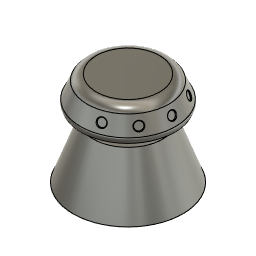
forme1 (Autodesk Fusion 360 design; units mm, degrees)
Autodesk Fusion 360 part; units mm, degrees
note: some values were not read from the file. Set by a fixed rule: which sketch regions a step uses.
sketch "Esquisse2" plane through (0, 0, 0) normal (0, 0, 1) x (1, 0, 0)
  line L0 (-70, 0) -> (-98.2998, 28.2688)
  line L1 (-98.2998, 28.2688) -> (-76.4677, 78.2688)
  line L2 (-76.4677, 78.2688) -> (0, 78.2688)
  line L3 (0, 78.2688) -> (0, 0)
  line L4 (-70, 0) -> (-110, -110)
  line L5 (-110, -110) -> (0, -110)
  line L6 (0, -110) -> (0, 0)
  dimension "d4" = 40
  dimension "d5" = 70
  dimension "d6" = 50
  dimension "d12" = 110
  constraint horizontal L2
  constraint coincident L3.end L6.end
  measures "d4" distance of L0.start L0.end
  measures "d5" distance of L3.end L0.start
  measures "d6" vertical distance of L0.end L1.end
  measures "d12" vertical distance of L0.start L4.end
revolve "Révolution1" add sketch "Esquisse2" angle 360 about axis through (0, 78.2688, 0) along (0, -1, 0)
fillet "Congé1" radius 10 1 edges at (-91.6476, 28.2688, 35.5467)
fillet "Congé2" radius 20 1 edges at (-71.293, 78.2688, 27.6519)
move_body "Déplacer1" bodies 1 to x (1, 0, 0) y (0, 1, 0) z (0, 0, 1) at (0, 110, 0)
hole "Perçage1" at (0, 161.3042, -88.2416) direction (0, -0.400157, 0.916446) diameter 15 depth 2 tip angle 180
fillet "Congé3" radius 1 2 edges at (-7.4998, 161.185, -87.9745) (7.4998, 161.185, -87.9745)
hole "Perçage2" at (72.2317, 161.4483, -50.5772) direction (-0.750709, -0.400157, 0.525652) diameter 15 depth 2 tip angle 180
hole "Perçage3" at (88.7236, 160.2003, 0) direction (-0.916446, -0.400157, 0) diameter 15 depth 2 tip angle 180
hole "Perçage4" at (72.9458, 159.452, 51.0772) direction (-0.750709, -0.400157, -0.525652) diameter 15 depth 2 tip angle 180
hole "Perçage5" at (30.3233, 160.3472, 83.3126) direction (-0.313443, -0.400157, -0.861178) diameter 15 depth 2 tip angle 180
fillet "Congé4" radius 1 2 edges at (68.4273, 159.3339, 57.0689) (77.0307, 159.3339, 44.7819)
fillet "Congé5" radius 1 2 edges at (23.185, 160.2283, 85.628) (37.2799, 160.2283, 80.4979)
fillet "Congé6" radius 1 2 edges at (88.4581, 160.0814, -7.4998) (88.4581, 160.0814, 7.4998)
fillet "Congé7" radius 1 2 edges at (67.7112, 161.3287, -56.5675) (76.3146, 161.3287, -44.2805)
